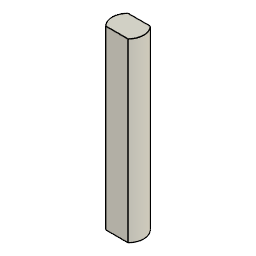
Wheel_Ax (Autodesk Fusion 360 design; units mm, degrees)
Autodesk Fusion 360 part; units mm, degrees
sketch "Sketch1" plane through (0, 0, 0) normal (0, 0, 1) x (1, 0, 0)
  line L0 (-3, 3) -> (3, 3)
  line L1 (3, -3) -> (-3, -3)
  line L2 (-3, 3) -> (3, -3) construction
  line L3 (3, 3) -> (-3, -3) construction
  arc A0 (-3, 3) -> (-3, -3) centre (0, 0) ccw
  arc A1 (3, -3) -> (3, 3) centre (0, 0) ccw
  dimension "d1" = 6
  dimension "d2" = 6
  constraint horizontal L0
  constraint horizontal L1
  constraint midpoint A0.centre L3
  constraint coincident A0.centre A1.centre
  constraint concentric A0 A1
  measures "d1" distance of L0.start L0.end
  measures "d2" distance of L0.start L1.end
extrude "Extrude1" add sketch "Sketch1" along normal blind 47.5
equation "d3 = 35.4 mm + 8 mm + 4.1 mm"
